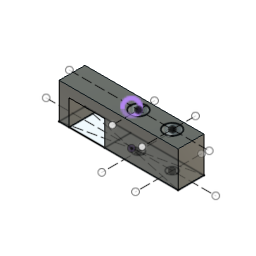
Power_plug_holder v3 (Autodesk Fusion 360 design; units mm, degrees)
Autodesk Fusion 360 part; units mm, degrees
sketch "Skizze1" plane through (0, 0, 0) normal (0, 0, 1) x (1, 0, 0)
  line L0 (15, -3.25) -> (-15, -3.25)
  line L1 (-15, -3.25) -> (-15, 3.25)
  line L2 (-15, 3.25) -> (15, 3.25)
  line L3 (15, 3.25) -> (15, -3.25)
  line L4 (15, -3.25) -> (-15, 3.25) construction
  line L5 (-15, -3.25) -> (15, 3.25) construction
  line L6 (-21.7851, 0.25) -> (21, 0.25) construction
  line L7 (10, 7.6042) -> (10, -9) construction
  line L8 (1.5, 8) -> (1.5, -9) construction
  line L9 (-3.5, 3.25) -> (-3.5, -3.25)
  line L10 (-12.5, 3.25) -> (-12.5, -3.25)
  circle A0 centre (10, 0.25) radius 1.25
  circle A1 centre (1.5, 0.25) radius 1.25
  dimension "d1" = 6.5
  dimension "d2" = 30
  dimension "d3" = 3
  dimension "d4" = 5
  dimension "d5" = 8.5
  dimension "d6" = 9
  dimension "d7" = 2.5
  dimension "d8" = 2.5
  dimension "d9" = 2.5
  constraint horizontal L0
  constraint perpendicular L0 L1
  constraint parallel L0 L2
  constraint parallel L1 L3
  constraint coincident L4 origin
  constraint coincident L5 origin
  constraint perpendicular L3 L6
  constraint vertical L7
  constraint vertical L8
  constraint coincident L2 L9.start
  constraint coincident L0 L9.end
  constraint perpendicular L0 L9
  constraint coincident L2 L10.start
  constraint coincident L0 L10.end
  constraint perpendicular L0 L10
  constraint coincident L6 A0.centre
  constraint coincident L7 A0.centre
  constraint coincident L8 A1.centre
  constraint coincident L6 A1.centre
  measures "d1" distance of L0 L2
  measures "d2" distance of L1 L3
  measures "d3" distance of L2 L6
  measures "d4" distance of L3 L7
  measures "d5" distance of L7 L8
  measures "d6" distance of L9 L10
  measures "d7" distance of L1 L10
  measures "d8" diameter of A1
  measures "d9" diameter of A0
extrude "Extrusion1" add sketch "Skizze1" along normal blind 9
extrude "Extrusion2" cut sketch "Skizze1" along normal blind 6.4 contours L0 L2 L9 L10
sketch "Skizze2" plane through (0, 0, 9) normal (0, 0, 1) x (-1, 0, 0)
  circle A0 centre (-10, -0.25) radius 1.25
  circle A1 centre (-1.5, -0.25) radius 1.25
  line L0 (-15, -3.25) -> (15, -3.25)
  line L1 (15, -3.25) -> (15, 3.25)
  line L2 (15, 3.25) -> (-15, 3.25)
  line L3 (-15, 3.25) -> (-15, -3.25)
  line L4 (15.9329, -0.25) -> (-19.3468, -0.25) construction
  line L5 (-10, -6.1266) -> (-10, 7.3493) construction
  line L6 (-1.5, 6.35) -> (-1.5, -4.2794) construction
  circle A2 centre (-1.5, -0.25) radius 2
  circle A3 centre (-10, -0.25) radius 2
  dimension "d14" = 0.25
  dimension "d15" = 10
  dimension "d16" = 8.5
  dimension "d17" = 4
  dimension "d18" = 4
  constraint perpendicular L3 L4
  constraint vertical L5
  constraint perpendicular L2 L6
  constraint concentric A1 A2
  constraint concentric A0 A3
  measures "d14" distance of L4 origin
  measures "d15" distance of L5 origin
  measures "d16" distance of L5 L6
  measures "d17" diameter of A3
  measures "d18" diameter of A2
extrude "Extrusion3" cut sketch "Skizze2" against normal blind 4 contours A2
extrude "Extrusion4" cut sketch "Skizze2" against normal blind 4 contours A3
